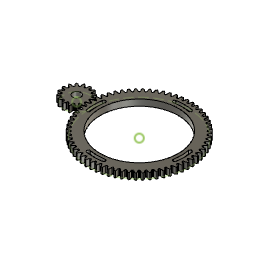
gear use (Autodesk Fusion 360 design; units mm, degrees)
description: Spur Gear; Module: 1.0; Num Teeth: 16; Pressure Angle: 20.0; Backlash: 0.15 mm
description: Spur Gear; Module: 1.0; Num Teeth: 64; Pressure Angle: 20.0; Backlash: 0.15 mm
Autodesk Fusion 360 part; units mm, degrees
(part 1 of 6)
sketch "Sketch1" plane through (0, 0, 0) normal (0, 0, 1) x (1, 0, 0) in component "Spur Gear (16 teeth)"
  circle A0 centre (0, 0) radius 6.7492
  circle A1 centre (0, 0) radius 2.6
  dimension "d41" = 5.2
  measures "d41" diameter of A1
extrude "Extrude1" add sketch "Sketch1" along normal blind 4 makes body 1 in component "Spur Gear (16 teeth)"
sketch "Sketch2" plane through (0, 0, 0) normal (0, 0, 1) x (1, 0, 0) in component "Spur Gear (16 teeth)"
  spline S0 degree 5 poles (7.4734, -0.8132) (7.4777, -0.8137) (7.4864, -0.8145) (7.4993, -0.8154) (7.5167, -0.8158) (7.5384, -0.8154) (7.5601, -0.8143) (7.5819, -0.8127) (7.6037, -0.811) (7.6256, -0.809) (7.6474, -0.8069) (7.6693, -0.8046) (7.6912, -0.8019) (7.7131, -0.799) (7.735, -0.7957) (7.7569, -0.7921) (7.7788, -0.7882) (7.8008, -0.7841) (7.8227, -0.7797) (7.8446, -0.7752) (7.8666, -0.7705) (7.8885, -0.7656) (7.9105, -0.7605) (7.9324, -0.7552) (7.9544, -0.7497) (7.9763, -0.7439) (7.9983, -0.738) (8.0202, -0.7318) (8.0422, -0.7255) (8.0641, -0.719) (8.0861, -0.7124) (8.108, -0.7055) (8.1299, -0.6985) (8.1518, -0.6913) (8.1737, -0.6839) (8.1956, -0.6764) (8.2175, -0.6687) (8.2394, -0.6608) (8.2613, -0.6528) (8.2831, -0.6446) (8.305, -0.6362) (8.3268, -0.6277) (8.3487, -0.619) (8.3705, -0.6102) (8.3923, -0.6012) (8.4141, -0.592) (8.4358, -0.5827) (8.4576, -0.5733) (8.4794, -0.5637) (8.5011, -0.5539) (8.5228, -0.544) (8.5445, -0.534) (8.5662, -0.5238) (8.5878, -0.5135) (8.6095, -0.503) (8.6311, -0.4924) (8.6527, -0.4816) (8.6743, -0.4707) (8.6958, -0.4596) (8.7174, -0.4485) (8.7389, -0.4371) (8.7604, -0.4257) (8.7819, -0.4141) (8.8033, -0.4023) (8.8248, -0.3905) (8.8462, -0.3784) (8.8676, -0.3663) (8.8889, -0.354) (8.9102, -0.3416) (8.9315, -0.3291) (8.9528, -0.3164) (8.9698, -0.3061) (8.9826, -0.2984) (8.9911, -0.2932) (8.9953, -0.2906) knots 0 0 0 0 0 0 0.01428571 0.02857143 0.04285714 0.05714286 0.07142857 0.08571429 0.1 0.11428571 0.12857143 0.14285714 0.15714286 0.17142857 0.18571429 0.2 0.21428571 0.22857143 0.24285714 0.25714286 0.27142857 0.28571429 0.3 0.31428571 0.32857143 0.34285714 0.35714286 0.37142857 0.38571429 0.4 0.41428571 0.42857143 0.44285714 0.45714286 0.47142857 0.48571429 0.5 0.51428571 0.52857143 0.54285714 0.55714286 0.57142857 0.58571429 0.6 0.61428571 0.62857143 0.64285714 0.65714286 0.67142857 0.68571429 0.7 0.71428571 0.72857143 0.74285714 0.75714286 0.77142857 0.78571429 0.8 0.81428571 0.82857143 0.84285714 0.85714286 0.87142857 0.88571429 0.9 0.91428571 0.92857143 0.94285714 0.95714286 0.97142857 0.98571429 1 1 1 1 1 1
  spline S1 degree 5 poles (7.4734, 0.8132) (7.4777, 0.8137) (7.4864, 0.8145) (7.4993, 0.8154) (7.5167, 0.8158) (7.5384, 0.8154) (7.5601, 0.8143) (7.5819, 0.8127) (7.6037, 0.811) (7.6256, 0.809) (7.6474, 0.8069) (7.6693, 0.8046) (7.6912, 0.8019) (7.7131, 0.799) (7.735, 0.7957) (7.7569, 0.7921) (7.7788, 0.7882) (7.8008, 0.7841) (7.8227, 0.7797) (7.8446, 0.7752) (7.8666, 0.7705) (7.8885, 0.7656) (7.9105, 0.7605) (7.9324, 0.7552) (7.9544, 0.7497) (7.9763, 0.7439) (7.9983, 0.738) (8.0202, 0.7318) (8.0422, 0.7255) (8.0641, 0.719) (8.0861, 0.7124) (8.108, 0.7055) (8.1299, 0.6985) (8.1518, 0.6913) (8.1737, 0.6839) (8.1956, 0.6764) (8.2175, 0.6687) (8.2394, 0.6608) (8.2613, 0.6528) (8.2831, 0.6446) (8.305, 0.6362) (8.3268, 0.6277) (8.3487, 0.619) (8.3705, 0.6102) (8.3923, 0.6012) (8.4141, 0.592) (8.4358, 0.5827) (8.4576, 0.5733) (8.4794, 0.5637) (8.5011, 0.5539) (8.5228, 0.544) (8.5445, 0.534) (8.5662, 0.5238) (8.5878, 0.5135) (8.6095, 0.503) (8.6311, 0.4924) (8.6527, 0.4816) (8.6743, 0.4707) (8.6958, 0.4596) (8.7174, 0.4485) (8.7389, 0.4371) (8.7604, 0.4257) (8.7819, 0.4141) (8.8033, 0.4023) (8.8248, 0.3905) (8.8462, 0.3784) (8.8676, 0.3663) (8.8889, 0.354) (8.9102, 0.3416) (8.9315, 0.3291) (8.9528, 0.3164) (8.9698, 0.3061) (8.9826, 0.2984) (8.9911, 0.2932) (8.9953, 0.2906) knots 0 0 0 0 0 0 0.01428571 0.02857143 0.04285714 0.05714286 0.07142857 0.08571429 0.1 0.11428571 0.12857143 0.14285714 0.15714286 0.17142857 0.18571429 0.2 0.21428571 0.22857143 0.24285714 0.25714286 0.27142857 0.28571429 0.3 0.31428571 0.32857143 0.34285714 0.35714286 0.37142857 0.38571429 0.4 0.41428571 0.42857143 0.44285714 0.45714286 0.47142857 0.48571429 0.5 0.51428571 0.52857143 0.54285714 0.55714286 0.57142857 0.58571429 0.6 0.61428571 0.62857143 0.64285714 0.65714286 0.67142857 0.68571429 0.7 0.71428571 0.72857143 0.74285714 0.75714286 0.77142857 0.78571429 0.8 0.81428571 0.82857143 0.84285714 0.85714286 0.87142857 0.88571429 0.9 0.91428571 0.92857143 0.94285714 0.95714286 0.97142857 0.98571429 1 1 1 1 1 1
  arc A0 (8.9953, -0.2906) -> (8.9953, 0.2906) centre (0, 0) ccw
  line L0 (6.6997, -0.7301) -> (7.4734, -0.8132)
  line L1 (6.6997, 0.7301) -> (7.4734, 0.8132)
  line L2 (6.6997, -0.7301) -> (6.6997, 0.7301)
  point P0 (7.58, -0.8128)
  point P1 (7.6876, -0.8023)
  point P2 (7.7958, -0.785)
  point P3 (7.9045, -0.7619)
  point P4 (8.0135, -0.7337)
  point P5 (8.1227, -0.7008)
  point P6 (8.2321, -0.6634)
  point P7 (8.3415, -0.6218)
  point P8 (8.4509, -0.5762)
  point P9 (8.5603, -0.5266)
  point P10 (8.6694, -0.4731)
  point P11 (8.7784, -0.4159)
  point P12 (8.887, -0.3551)
  point P13 (7.58, 0.8128)
  point P14 (7.6876, 0.8023)
  point P15 (7.7958, 0.785)
  point P16 (7.9045, 0.7619)
  point P17 (8.0135, 0.7337)
  point P18 (8.1227, 0.7008)
  point P19 (8.2321, 0.6634)
  point P20 (8.3415, 0.6218)
  point P21 (8.4509, 0.5762)
  point P22 (8.5603, 0.5266)
  point P23 (8.6694, 0.4731)
  point P24 (8.7784, 0.4159)
  point P25 (8.887, 0.3551)
extrude "Extrude2" add sketch "Sketch2" along normal blind 4 bodies 1 in component "Spur Gear (16 teeth)"
fillet "Fillet1" radius 0.5 2 edges at (6.7095, -0.7312, 2) (6.7095, 0.7312, 2) on bodies 1 in component "Spur Gear (16 teeth)"
pattern_circular "C-Pattern1" count 16 over 360 about axis through (0, 0, 0) along (0, 0, 1) of "Extrude2", "Fillet1" in component "Spur Gear (16 teeth)"
sketch "Sketch3" plane through (0, 0, 0) normal (0, 0, 1) x (1, 0, 0) in component "Spur Gear (16 teeth)"
  circle A0 centre (0, 0) radius 8 construction
sketch "Sketch1 (2)" plane through (0, 0, 0) normal (0, 0, 1) x (1, 0, 0) in component "Spur Gear (64 teeth)"
  circle A0 centre (0, 0) radius 30.7492
  circle A1 centre (0, 0) radius 25
extrude "Extrude1'" add sketch "Sketch1 (2)" along normal blind 4 separate body makes body 2 in component "Spur Gear (64 teeth)"
sketch "Sketch2 (2)" plane through (0, 0, 0) normal (0, 0, 1) x (1, 0, 0) in component "Spur Gear (64 teeth)"
  spline S0 degree 5 poles (30.0481, -1.1507) (30.0566, -1.1507) (30.0736, -1.1505) (30.0991, -1.1502) (30.1331, -1.1493) (30.1756, -1.1475) (30.2181, -1.1451) (30.2606, -1.1421) (30.3031, -1.1385) (30.3456, -1.1344) (30.3881, -1.1298) (30.4306, -1.1247) (30.4731, -1.1193) (30.5156, -1.1135) (30.5581, -1.1074) (30.6006, -1.101) (30.643, -1.0942) (30.6855, -1.0872) (30.728, -1.0798) (30.7704, -1.0722) (30.8128, -1.0642) (30.8553, -1.056) (30.8977, -1.0475) (30.9401, -1.0388) (30.9825, -1.0298) (31.0249, -1.0205) (31.0672, -1.011) (31.1096, -1.0012) (31.1519, -0.9913) (31.1943, -0.981) (31.2366, -0.9706) (31.2789, -0.9599) (31.3212, -0.949) (31.3635, -0.9378) (31.4057, -0.9265) (31.448, -0.9149) (31.4902, -0.9032) (31.5324, -0.8912) (31.5746, -0.879) (31.6168, -0.8666) (31.659, -0.854) (31.7011, -0.8413) (31.7433, -0.8283) (31.7854, -0.8151) (31.8275, -0.8017) (31.8696, -0.7882) (31.9116, -0.7744) (31.9537, -0.7605) (31.9957, -0.7464) (32.0377, -0.7321) (32.0797, -0.7176) (32.1216, -0.7029) (32.1636, -0.6881) (32.2055, -0.6731) (32.2474, -0.6579) (32.2893, -0.6425) (32.3312, -0.627) (32.373, -0.6113) (32.4149, -0.5954) (32.4567, -0.5793) (32.4984, -0.5631) (32.5402, -0.5467) (32.5819, -0.5302) (32.6237, -0.5135) (32.6654, -0.4966) (32.707, -0.4796) (32.7487, -0.4624) (32.7903, -0.445) (32.8319, -0.4275) (32.8735, -0.4098) (32.915, -0.392) (32.9483, -0.3776) (32.9732, -0.3667) (32.9898, -0.3594) (32.9981, -0.3558) knots 0 0 0 0 0 0 0.01428571 0.02857143 0.04285714 0.05714286 0.07142857 0.08571429 0.1 0.11428571 0.12857143 0.14285714 0.15714286 0.17142857 0.18571429 0.2 0.21428571 0.22857143 0.24285714 0.25714286 0.27142857 0.28571429 0.3 0.31428571 0.32857143 0.34285714 0.35714286 0.37142857 0.38571429 0.4 0.41428571 0.42857143 0.44285714 0.45714286 0.47142857 0.48571429 0.5 0.51428571 0.52857143 0.54285714 0.55714286 0.57142857 0.58571429 0.6 0.61428571 0.62857143 0.64285714 0.65714286 0.67142857 0.68571429 0.7 0.71428571 0.72857143 0.74285714 0.75714286 0.77142857 0.78571429 0.8 0.81428571 0.82857143 0.84285714 0.85714286 0.87142857 0.88571429 0.9 0.91428571 0.92857143 0.94285714 0.95714286 0.97142857 0.98571429 1 1 1 1 1 1
  spline S1 degree 5 poles (30.0481, 1.1507) (30.0566, 1.1507) (30.0736, 1.1505) (30.0991, 1.1502) (30.1331, 1.1493) (30.1756, 1.1475) (30.2181, 1.1451) (30.2606, 1.1421) (30.3031, 1.1385) (30.3456, 1.1344) (30.3881, 1.1298) (30.4306, 1.1247) (30.4731, 1.1193) (30.5156, 1.1135) (30.5581, 1.1074) (30.6006, 1.101) (30.643, 1.0942) (30.6855, 1.0872) (30.728, 1.0798) (30.7704, 1.0722) (30.8128, 1.0642) (30.8553, 1.056) (30.8977, 1.0475) (30.9401, 1.0388) (30.9825, 1.0298) (31.0249, 1.0205) (31.0672, 1.011) (31.1096, 1.0012) (31.1519, 0.9913) (31.1943, 0.981) (31.2366, 0.9706) (31.2789, 0.9599) (31.3212, 0.949) (31.3635, 0.9378) (31.4057, 0.9265) (31.448, 0.9149) (31.4902, 0.9032) (31.5324, 0.8912) (31.5746, 0.879) (31.6168, 0.8666) (31.659, 0.854) (31.7011, 0.8413) (31.7433, 0.8283) (31.7854, 0.8151) (31.8275, 0.8017) (31.8696, 0.7882) (31.9116, 0.7744) (31.9537, 0.7605) (31.9957, 0.7464) (32.0377, 0.7321) (32.0797, 0.7176) (32.1216, 0.7029) (32.1636, 0.6881) (32.2055, 0.6731) (32.2474, 0.6579) (32.2893, 0.6425) (32.3312, 0.627) (32.373, 0.6113) (32.4149, 0.5954) (32.4567, 0.5793) (32.4984, 0.5631) (32.5402, 0.5467) (32.5819, 0.5302) (32.6237, 0.5135) (32.6654, 0.4966) (32.707, 0.4796) (32.7487, 0.4624) (32.7903, 0.445) (32.8319, 0.4275) (32.8735, 0.4098) (32.915, 0.392) (32.9483, 0.3776) (32.9732, 0.3667) (32.9898, 0.3594) (32.9981, 0.3558) knots 0 0 0 0 0 0 0.01428571 0.02857143 0.04285714 0.05714286 0.07142857 0.08571429 0.1 0.11428571 0.12857143 0.14285714 0.15714286 0.17142857 0.18571429 0.2 0.21428571 0.22857143 0.24285714 0.25714286 0.27142857 0.28571429 0.3 0.31428571 0.32857143 0.34285714 0.35714286 0.37142857 0.38571429 0.4 0.41428571 0.42857143 0.44285714 0.45714286 0.47142857 0.48571429 0.5 0.51428571 0.52857143 0.54285714 0.55714286 0.57142857 0.58571429 0.6 0.61428571 0.62857143 0.64285714 0.65714286 0.67142857 0.68571429 0.7 0.71428571 0.72857143 0.74285714 0.75714286 0.77142857 0.78571429 0.8 0.81428571 0.82857143 0.84285714 0.85714286 0.87142857 0.88571429 0.9 0.91428571 0.92857143 0.94285714 0.95714286 0.97142857 0.98571429 1 1 1 1 1 1
  arc A0 (32.9981, -0.3558) -> (32.9981, 0.3558) centre (0, 0) ccw
  line L0 (30.0481, 1.1507) -> (30.0481, -1.1507)
  point P0 (30.2579, -1.1422)
  point P1 (30.4681, -1.1198)
  point P2 (30.6787, -1.0883)
  point P3 (30.8894, -1.0491)
  point P4 (31.1004, -1.0033)
  point P5 (31.3114, -0.9515)
  point P6 (31.5224, -0.894)
  point P7 (31.7335, -0.8313)
  point P8 (31.9445, -0.7635)
  point P9 (32.1555, -0.6909)
  point P10 (32.3664, -0.6137)
  point P11 (32.5771, -0.5321)
  point P12 (32.7877, -0.446)
  point P13 (30.2579, 1.1422)
  point P14 (30.4681, 1.1198)
  point P15 (30.6787, 1.0883)
  point P16 (30.8894, 1.0491)
  point P17 (31.1004, 1.0033)
  point P18 (31.3114, 0.9515)
  point P19 (31.5224, 0.894)
  point P20 (31.7335, 0.8313)
  point P21 (31.9445, 0.7635)
  point P22 (32.1555, 0.6909)
  point P23 (32.3664, 0.6137)
  point P24 (32.5771, 0.5321)
  point P25 (32.7877, 0.446)
extrude "Extrude2'" add sketch "Sketch2 (2)" along normal blind 4 bodies 2 in component "Spur Gear (64 teeth)"
fillet "Fillet1'" radius 0.5 2 edges at (30.7303, 1.0794, 2) (30.7303, -1.0794, 2) on bodies 2 in component "Spur Gear (64 teeth)"
pattern_circular "C-Pattern1'" count 64 over 360 about axis through (0, 0, -0.0002) along (0, 0, 1) of "Extrude2'", "Fillet1'" in component "Spur Gear (64 teeth)"
sketch "Sketch3 (2)" plane through (0, 0, 0) normal (0, 0, 1) x (1, 0, 0) in component "Spur Gear (64 teeth)"
  circle A0 centre (0, 0) radius 32 construction
sketch "Sketch1 (3)" plane through (0, 0, 0) normal (0, 0, 1) x (1, 0, 0)
  circle A0 centre (0, 0) radius 10
  circle A1 centre (40, 0) radius 33.936
  line L0 (19.6927, 27.1894) -> (-5.984, 8.012)
  line L1 (0, 0) -> (40, 0) construction
  line L2 (19.6927, -27.1894) -> (-5.984, -8.012)
  point P0 (40, 0)
  constraint coincident A0.centre L1.start
  constraint tangent A1 L0
  constraint tangent A0 L0
  constraint coincident P0 A1.centre
  constraint coincident A1 L0.start
  constraint coincident A0 L0.end
  constraint symmetric L0.start L1 L2.start
  constraint symmetric L0.end L1 L2.end
sketch "Sketch3 (3)" plane through (0, 0, 4) normal (0, 0, 1) x (-1, 0, 0)
  arc A0 (-70.5976, 3.0494) -> (-70.6059, 2.9651) centre (-40, 0) ccw
  spline S0 degree 3 poles (-71.0146, 2.5213) (-70.9505, 2.5329) (-70.8893, 2.5569) (-70.7796, 2.627) (-70.7321, 2.6724) (-70.6698, 2.7609) (-70.6497, 2.7992) (-70.6197, 2.88) (-70.6101, 2.9222) (-70.6059, 2.9651) knots 0 0 0 0 0.019532 0.019532 0.039064 0.039064 0.051994 0.051994 0.064924 0.064924 0.064924 0.064924
  spline S1 degree 5 poles (-71.0146, 2.5213) (-71.0164, 2.521) (-71.0267, 2.5191) (-71.0456, 2.5157) (-71.0731, 2.5105) (-71.1091, 2.5037) (-71.1519, 2.4953) (-71.1947, 2.4867) (-71.2374, 2.4779) (-71.2802, 2.4688) (-71.323, 2.4596) (-71.3657, 2.4501) (-71.4085, 2.4404) (-71.4512, 2.4305) (-71.494, 2.4204) (-71.5367, 2.4101) (-71.5795, 2.3996) (-71.6222, 2.3889) (-71.6649, 2.3779) (-71.7076, 2.3668) (-71.7503, 2.3555) (-71.793, 2.3441) (-71.8357, 2.3324) (-71.8784, 2.3205) (-71.921, 2.3085) (-71.9637, 2.2962) (-72.0063, 2.2838) (-72.049, 2.2712) (-72.0916, 2.2585) (-72.1342, 2.2455) (-72.1768, 2.2324) (-72.2194, 2.2191) (-72.262, 2.2056) (-72.3045, 2.192) (-72.3471, 2.1781) (-72.3896, 2.1641) (-72.4321, 2.15) (-72.4746, 2.1357) (-72.5171, 2.1212) (-72.5596, 2.1065) (-72.6021, 2.0917) (-72.6446, 2.0767) (-72.687, 2.0616) (-72.7294, 2.0463) (-72.7718, 2.0308) (-72.8142, 2.0152) (-72.8566, 1.9994) (-72.8905, 1.9866) (-72.9159, 1.977) (-72.9328, 1.9705) (-72.9413, 1.9673) knots 0.354152 0.354152 0.354152 0.354152 0.354152 0.354152 0.357143 0.371429 0.385714 0.4 0.414286 0.428571 0.442857 0.457143 0.471429 0.485714 0.5 0.514286 0.528571 0.542857 0.557143 0.571429 0.585714 0.6 0.614286 0.628571 0.642857 0.657143 0.671429 0.685714 0.7 0.714286 0.728571 0.742857 0.757143 0.771429 0.785714 0.8 0.814286 0.828571 0.842857 0.857143 0.871429 0.885714 0.9 0.914286 0.928571 0.942857 0.957143 0.971429 0.985714 1 1 1 1 1 1
  arc A1 (-72.9413, 1.9673) -> (-72.9761, 1.2566) centre (-40, 0) ccw
  spline S2 degree 5 poles (-72.9761, 1.2566) (-72.968, 1.2525) (-72.9517, 1.2445) (-72.9274, 1.2324) (-72.8949, 1.2164) (-72.8543, 1.1966) (-72.8136, 1.1769) (-72.7729, 1.1573) (-72.7322, 1.138) (-72.6914, 1.1188) (-72.6506, 1.0997) (-72.6098, 1.0808) (-72.5689, 1.0621) (-72.5281, 1.0435) (-72.4872, 1.0251) (-72.4462, 1.0069) (-72.4052, 0.9888) (-72.3642, 0.9709) (-72.3232, 0.9531) (-72.2822, 0.9356) (-72.2411, 0.9182) (-72.2, 0.901) (-72.1588, 0.8839) (-72.1176, 0.867) (-72.0764, 0.8503) (-72.0352, 0.8338) (-71.9939, 0.8175) (-71.9527, 0.8013) (-71.9113, 0.7854) (-71.87, 0.7696) (-71.8286, 0.754) (-71.7872, 0.7386) (-71.7458, 0.7234) (-71.7044, 0.7083) (-71.6629, 0.6935) (-71.6214, 0.6789) (-71.5799, 0.6644) (-71.5383, 0.6502) (-71.4967, 0.6362) (-71.4551, 0.6224) (-71.4135, 0.6088) (-71.3718, 0.5954) (-71.3302, 0.5822) (-71.2885, 0.5692) (-71.2467, 0.5565) (-71.205, 0.544) (-71.1698, 0.5336) (-71.143, 0.5259) (-71.1245, 0.5206) (-71.1144, 0.5177) (-71.1126, 0.5172) knots -1 -1 -1 -1 -1 -1 -0.985714 -0.971429 -0.957143 -0.942857 -0.928571 -0.914286 -0.9 -0.885714 -0.871429 -0.857143 -0.842857 -0.828571 -0.814286 -0.8 -0.785714 -0.771429 -0.757143 -0.742857 -0.728571 -0.714286 -0.7 -0.685714 -0.671429 -0.657143 -0.642857 -0.628571 -0.614286 -0.6 -0.585714 -0.571429 -0.557143 -0.542857 -0.528571 -0.514286 -0.5 -0.485714 -0.471429 -0.457143 -0.442857 -0.428571 -0.414286 -0.4 -0.385714 -0.371429 -0.357143 -0.354152 -0.354152 -0.354152 -0.354152 -0.354152 -0.354152
  spline S3 degree 3 poles (-70.7492, 0.0357) (-70.7491, 0.1008) (-70.7617, 0.1653) (-70.811, 0.2858) (-70.8472, 0.3407) (-70.9231, 0.4178) (-70.9572, 0.4444) (-71.0314, 0.4884) (-71.0712, 0.5054) (-71.1126, 0.5172) knots 0 0 0 0 0.019532 0.019532 0.039064 0.039064 0.051994 0.051994 0.064924 0.064924 0.064924 0.064924
  arc A2 (-70.7492, 0.0357) -> (-70.7492, -0.0491) centre (-40, 0) ccw
  spline S4 degree 3 poles (-71.1124, -0.5308) (-71.0498, -0.513) (-70.9912, -0.4831) (-70.8889, -0.4026) (-70.846, -0.3527) (-70.7928, -0.2586) (-70.7765, -0.2185) (-70.7546, -0.1351) (-70.7491, -0.0922) (-70.7492, -0.0491) knots 0 0 0 0 0.019532 0.019532 0.039064 0.039064 0.051994 0.051994 0.064924 0.064924 0.064924 0.064924
  spline S5 degree 5 poles (-71.1124, -0.5308) (-71.1141, -0.5313) (-71.1242, -0.5342) (-71.1427, -0.5395) (-71.1696, -0.5472) (-71.2047, -0.5576) (-71.2465, -0.5701) (-71.2882, -0.5829) (-71.3299, -0.5959) (-71.3716, -0.6091) (-71.4132, -0.6225) (-71.4549, -0.6361) (-71.4965, -0.6499) (-71.538, -0.664) (-71.5796, -0.6782) (-71.6211, -0.6927) (-71.6626, -0.7073) (-71.7041, -0.7222) (-71.7455, -0.7372) (-71.7869, -0.7524) (-71.8283, -0.7679) (-71.8697, -0.7835) (-71.911, -0.7993) (-71.9523, -0.8153) (-71.9936, -0.8314) (-72.0348, -0.8478) (-72.0761, -0.8643) (-72.1173, -0.8811) (-72.1584, -0.8979) (-72.1996, -0.915) (-72.2407, -0.9322) (-72.2817, -0.9497) (-72.3228, -0.9672) (-72.3638, -0.985) (-72.4048, -1.0029) (-72.4458, -1.021) (-72.4867, -1.0393) (-72.5276, -1.0577) (-72.5685, -1.0763) (-72.6093, -1.095) (-72.6501, -1.1139) (-72.6909, -1.133) (-72.7317, -1.1522) (-72.7724, -1.1716) (-72.8131, -1.1912) (-72.8537, -1.2109) (-72.8944, -1.2308) (-72.9268, -1.2468) (-72.9512, -1.2588) (-72.9674, -1.2669) (-72.9755, -1.271) knots 0.354152 0.354152 0.354152 0.354152 0.354152 0.354152 0.357143 0.371429 0.385714 0.4 0.414286 0.428571 0.442857 0.457143 0.471429 0.485714 0.5 0.514286 0.528571 0.542857 0.557143 0.571429 0.585714 0.6 0.614286 0.628571 0.642857 0.657143 0.671429 0.685714 0.7 0.714286 0.728571 0.742857 0.757143 0.771429 0.785714 0.8 0.814286 0.828571 0.842857 0.857143 0.871429 0.885714 0.9 0.914286 0.928571 0.942857 0.957143 0.971429 0.985714 1 1 1 1 1 1
  arc A3 (-72.9755, -1.271) -> (-72.9404, -1.9817) centre (-40, 0) ccw
  spline S6 degree 5 poles (-72.9404, -1.9817) (-72.932, -1.9849) (-72.915, -1.9914) (-72.8896, -2.001) (-72.8557, -2.0137) (-72.8133, -2.0295) (-72.7709, -2.0451) (-72.7285, -2.0605) (-72.6861, -2.0758) (-72.6436, -2.091) (-72.6012, -2.1059) (-72.5587, -2.1207) (-72.5162, -2.1354) (-72.4737, -2.1498) (-72.4312, -2.1641) (-72.3887, -2.1783) (-72.3461, -2.1922) (-72.3036, -2.206) (-72.261, -2.2197) (-72.2184, -2.2331) (-72.1758, -2.2464) (-72.1332, -2.2595) (-72.0906, -2.2725) (-72.048, -2.2852) (-72.0053, -2.2978) (-71.9627, -2.3102) (-71.92, -2.3224) (-71.8773, -2.3344) (-71.8347, -2.3463) (-71.792, -2.3579) (-71.7493, -2.3694) (-71.7066, -2.3807) (-71.6639, -2.3918) (-71.6211, -2.4027) (-71.5784, -2.4133) (-71.5357, -2.4238) (-71.4929, -2.4341) (-71.4502, -2.4442) (-71.4074, -2.4541) (-71.3647, -2.4638) (-71.3219, -2.4732) (-71.2791, -2.4825) (-71.2364, -2.4915) (-71.1936, -2.5003) (-71.1508, -2.5089) (-71.108, -2.5173) (-71.072, -2.5241) (-71.0445, -2.5292) (-71.0256, -2.5326) (-71.0153, -2.5345) (-71.0135, -2.5348) knots -1 -1 -1 -1 -1 -1 -0.985714 -0.971429 -0.957143 -0.942857 -0.928571 -0.914286 -0.9 -0.885714 -0.871429 -0.857143 -0.842857 -0.828571 -0.814286 -0.8 -0.785714 -0.771429 -0.757143 -0.742857 -0.728571 -0.714286 -0.7 -0.685714 -0.671429 -0.657143 -0.642857 -0.628571 -0.614286 -0.6 -0.585714 -0.571429 -0.557143 -0.542857 -0.528571 -0.514286 -0.5 -0.485714 -0.471429 -0.457143 -0.442857 -0.428571 -0.414286 -0.4 -0.385714 -0.371429 -0.357143 -0.354152 -0.354152 -0.354152 -0.354152 -0.354152 -0.354152
  spline S7 degree 3 poles (-70.6046, -2.9785) (-70.6109, -2.9137) (-70.6298, -2.8507) (-70.6907, -2.7356) (-70.7321, -2.6845) (-70.8152, -2.6153) (-70.8517, -2.5921) (-70.9298, -2.5556) (-70.9711, -2.5425) (-71.0135, -2.5348) knots 0 0 0 0 0.019532 0.019532 0.039064 0.039064 0.051994 0.051994 0.064924 0.064924 0.064924 0.064924
  arc A4 (-70.6046, -2.9785) -> (-70.5963, -3.0628) centre (-40, 0) ccw
  spline S8 degree 3 poles (-70.9105, -3.5778) (-70.85, -3.5539) (-70.7946, -3.5185) (-70.7007, -3.4283) (-70.6629, -3.3745) (-70.6191, -3.2755) (-70.6069, -3.234) (-70.5933, -3.1489) (-70.592, -3.1057) (-70.5963, -3.0628) knots 0 0 0 0 0.019532 0.019532 0.039064 0.039064 0.051994 0.051994 0.064924 0.064924 0.064924 0.064924
  spline S9 degree 5 poles (-70.9105, -3.5778) (-70.9122, -3.5785) (-70.922, -3.5823) (-70.9399, -3.5894) (-70.9658, -3.5998) (-70.9998, -3.6135) (-71.0401, -3.6301) (-71.0804, -3.6469) (-71.1206, -3.6639) (-71.1608, -3.6811) (-71.201, -3.6985) (-71.241, -3.7161) (-71.2811, -3.734) (-71.3211, -3.752) (-71.361, -3.7703) (-71.4009, -3.7887) (-71.4408, -3.8074) (-71.4806, -3.8262) (-71.5204, -3.8453) (-71.5601, -3.8645) (-71.5998, -3.8839) (-71.6394, -3.9035) (-71.679, -3.9233) (-71.7185, -3.9432) (-71.758, -3.9634) (-71.7975, -3.9837) (-71.8369, -4.0042) (-71.8762, -4.0248) (-71.9156, -4.0457) (-71.9548, -4.0667) (-71.994, -4.0879) (-72.0332, -4.1093) (-72.0723, -4.1308) (-72.1114, -4.1525) (-72.1505, -4.1743) (-72.1895, -4.1963) (-72.2284, -4.2185) (-72.2673, -4.2409) (-72.3062, -4.2634) (-72.345, -4.286) (-72.3837, -4.3089) (-72.4224, -4.3318) (-72.4611, -4.355) (-72.4997, -4.3783) (-72.5383, -4.4017) (-72.5768, -4.4253) (-72.6153, -4.449) (-72.6461, -4.4682) (-72.6691, -4.4826) (-72.6845, -4.4922) (-72.6922, -4.497) knots 0.354152 0.354152 0.354152 0.354152 0.354152 0.354152 0.357143 0.371429 0.385714 0.4 0.414286 0.428571 0.442857 0.457143 0.471429 0.485714 0.5 0.514286 0.528571 0.542857 0.557143 0.571429 0.585714 0.6 0.614286 0.628571 0.642857 0.657143 0.671429 0.685714 0.7 0.714286 0.728571 0.742857 0.757143 0.771429 0.785714 0.8 0.814286 0.828571 0.842857 0.857143 0.871429 0.885714 0.9 0.914286 0.928571 0.942857 0.957143 0.971429 0.985714 1 1 1 1 1 1
  arc A5 (-72.6922, -4.497) -> (-72.5876, -5.2009) centre (-40, 0) ccw
  spline S10 degree 5 poles (-72.5876, -5.2009) (-72.5788, -5.2033) (-72.5614, -5.208) (-72.5351, -5.2151) (-72.5001, -5.2245) (-72.4564, -5.236) (-72.4127, -5.2474) (-72.369, -5.2586) (-72.3252, -5.2696) (-72.2815, -5.2805) (-72.2378, -5.2913) (-72.1941, -5.3018) (-72.1503, -5.3122) (-72.1066, -5.3225) (-72.0629, -5.3325) (-72.0192, -5.3424) (-71.9755, -5.3522) (-71.9318, -5.3617) (-71.8881, -5.3711) (-71.8444, -5.3803) (-71.8007, -5.3894) (-71.757, -5.3983) (-71.7133, -5.4069) (-71.6697, -5.4155) (-71.626, -5.4238) (-71.5823, -5.432) (-71.5387, -5.4399) (-71.495, -5.4477) (-71.4514, -5.4553) (-71.4078, -5.4627) (-71.3642, -5.47) (-71.3206, -5.477) (-71.277, -5.4838) (-71.2334, -5.4905) (-71.1898, -5.4969) (-71.1462, -5.5032) (-71.1027, -5.5093) (-71.0592, -5.5151) (-71.0156, -5.5207) (-70.9721, -5.5262) (-70.9287, -5.5314) (-70.8852, -5.5364) (-70.8417, -5.5412) (-70.7983, -5.5458) (-70.7549, -5.5501) (-70.7115, -5.5543) (-70.675, -5.5575) (-70.6471, -5.5599) (-70.628, -5.5615) (-70.6175, -5.5623) (-70.6157, -5.5625) knots -1 -1 -1 -1 -1 -1 -0.985714 -0.971429 -0.957143 -0.942857 -0.928571 -0.914286 -0.9 -0.885714 -0.871429 -0.857143 -0.842857 -0.828571 -0.814286 -0.8 -0.785714 -0.771429 -0.757143 -0.742857 -0.728571 -0.714286 -0.7 -0.685714 -0.671429 -0.657143 -0.642857 -0.628571 -0.614286 -0.6 -0.585714 -0.571429 -0.557143 -0.542857 -0.528571 -0.514286 -0.5 -0.485714 -0.471429 -0.457143 -0.442857 -0.428571 -0.414286 -0.4 -0.385714 -0.371429 -0.357143 -0.354152 -0.354152 -0.354152 -0.354152 -0.354152 -0.354152
  spline S11 degree 3 poles (-70.1653, -5.9639) (-70.1779, -5.9) (-70.2029, -5.8392) (-70.2748, -5.7306) (-70.321, -5.6839) (-70.4105, -5.6231) (-70.4491, -5.6036) (-70.5304, -5.5749) (-70.5727, -5.5659) (-70.6157, -5.5625) knots 0 0 0 0 0.019532 0.019532 0.039064 0.039064 0.051994 0.051994 0.064924 0.064924 0.064924 0.064924
  arc A6 (-70.1653, -5.9639) -> (-70.1488, -6.047) centre (-40, 0) ccw
  spline S12 degree 3 poles (-70.411, -6.5903) (-70.3531, -6.5606) (-70.3015, -6.5199) (-70.2168, -6.421) (-70.1845, -6.3637) (-70.1506, -6.261) (-70.1425, -6.2185) (-70.1373, -6.1324) (-70.1403, -6.0892) (-70.1488, -6.047) knots 0 0 0 0 0.019532 0.019532 0.039064 0.039064 0.051994 0.051994 0.064924 0.064924 0.064924 0.064924
  spline S13 degree 5 poles (-70.411, -6.5903) (-70.4126, -6.5912) (-70.422, -6.5959) (-70.4391, -6.6047) (-70.4639, -6.6176) (-70.4964, -6.6346) (-70.5349, -6.6551) (-70.5733, -6.6757) (-70.6117, -6.6966) (-70.65, -6.7176) (-70.6882, -6.7389) (-70.7264, -6.7604) (-70.7645, -6.7821) (-70.8025, -6.804) (-70.8405, -6.8261) (-70.8784, -6.8483) (-70.9162, -6.8708) (-70.954, -6.8934) (-70.9917, -6.9163) (-71.0293, -6.9393) (-71.0669, -6.9625) (-71.1045, -6.9859) (-71.1419, -7.0095) (-71.1793, -7.0332) (-71.2166, -7.0571) (-71.2539, -7.0812) (-71.2911, -7.1055) (-71.3282, -7.1299) (-71.3653, -7.1545) (-71.4023, -7.1792) (-71.4393, -7.2042) (-71.4762, -7.2293) (-71.513, -7.2545) (-71.5498, -7.2799) (-71.5865, -7.3055) (-71.6231, -7.3313) (-71.6597, -7.3571) (-71.6963, -7.3832) (-71.7327, -7.4094) (-71.7691, -7.4358) (-71.8055, -7.4623) (-71.8417, -7.4889) (-71.8779, -7.5157) (-71.9141, -7.5427) (-71.9502, -7.5698) (-71.9862, -7.5971) (-72.0222, -7.6245) (-72.0509, -7.6465) (-72.0724, -7.6631) (-72.0868, -7.6742) (-72.0939, -7.6798) knots 0.354152 0.354152 0.354152 0.354152 0.354152 0.354152 0.357143 0.371429 0.385714 0.4 0.414286 0.428571 0.442857 0.457143 0.471429 0.485714 0.5 0.514286 0.528571 0.542857 0.557143 0.571429 0.585714 0.6 0.614286 0.628571 0.642857 0.657143 0.671429 0.685714 0.7 0.714286 0.728571 0.742857 0.757143 0.771429 0.785714 0.8 0.814286 0.828571 0.842857 0.857143 0.871429 0.885714 0.9 0.914286 0.928571 0.942857 0.957143 0.971429 0.985714 1 1 1 1 1 1
  arc A7 (-72.0939, -7.6798) -> (-71.9209, -8.37) centre (-40, 0) ccw
  spline S14 degree 5 poles (-71.9209, -8.37) (-71.912, -8.3715) (-71.8941, -8.3745) (-71.8673, -8.379) (-71.8316, -8.3849) (-71.7869, -8.3921) (-71.7423, -8.3991) (-71.6977, -8.406) (-71.6531, -8.4127) (-71.6085, -8.4192) (-71.5639, -8.4256) (-71.5194, -8.4319) (-71.4748, -8.4379) (-71.4303, -8.4438) (-71.3858, -8.4496) (-71.3414, -8.4551) (-71.2969, -8.4605) (-71.2525, -8.4658) (-71.2081, -8.4708) (-71.1637, -8.4757) (-71.1193, -8.4804) (-71.075, -8.485) (-71.0306, -8.4894) (-70.9863, -8.4936) (-70.9421, -8.4976) (-70.8978, -8.5014) (-70.8536, -8.5051) (-70.8094, -8.5085) (-70.7652, -8.5118) (-70.7211, -8.5149) (-70.677, -8.5178) (-70.6329, -8.5206) (-70.5888, -8.5231) (-70.5448, -8.5255) (-70.5008, -8.5276) (-70.4569, -8.5296) (-70.4129, -8.5313) (-70.369, -8.5329) (-70.3252, -8.5342) (-70.2813, -8.5354) (-70.2376, -8.5363) (-70.1938, -8.537) (-70.1501, -8.5375) (-70.1064, -8.5378) (-70.0628, -8.5379) (-70.0192, -8.5378) (-69.9825, -8.5375) (-69.9546, -8.5371) (-69.9354, -8.5368) (-69.9249, -8.5366) (-69.9231, -8.5366) knots -1 -1 -1 -1 -1 -1 -0.985714 -0.971429 -0.957143 -0.942857 -0.928571 -0.914286 -0.9 -0.885714 -0.871429 -0.857143 -0.842857 -0.828571 -0.814286 -0.8 -0.785714 -0.771429 -0.757143 -0.742857 -0.728571 -0.714286 -0.7 -0.685714 -0.671429 -0.657143 -0.642857 -0.628571 -0.614286 -0.6 -0.585714 -0.571429 -0.557143 -0.542857 -0.528571 -0.514286 -0.5 -0.485714 -0.471429 -0.457143 -0.442857 -0.428571 -0.414286 -0.4 -0.385714 -0.371429 -0.357143 -0.354152 -0.354152 -0.354152 -0.354152 -0.354152 -0.354152
  spline S15 degree 3 poles (-69.4355, -8.8919) (-69.4543, -8.8296) (-69.4851, -8.7715) (-69.5673, -8.6705) (-69.6178, -8.6285) (-69.7129, -8.5767) (-69.7532, -8.5611) (-69.837, -8.5406) (-69.88, -8.5358) (-69.9231, -8.5366) knots 0 0 0 0 0.019532 0.019532 0.039064 0.039064 0.051994 0.051994 0.064924 0.064924 0.064924 0.064924
  arc A8 (-69.4355, -8.8919) -> (-69.4109, -8.973) centre (-40, 0) ccw
  spline S16 degree 3 poles (-69.6186, -9.5394) (-69.5639, -9.5042) (-69.5165, -9.4586) (-69.4419, -9.3518) (-69.4154, -9.2917) (-69.3918, -9.1861) (-69.3878, -9.143) (-69.3911, -9.0569) (-69.3983, -9.0142) (-69.4109, -8.973) knots 0 0 0 0 0.019532 0.019532 0.039064 0.039064 0.051994 0.051994 0.064924 0.064924 0.064924 0.064924
  spline S17 degree 5 poles (-69.6186, -9.5394) (-69.6201, -9.5404) (-69.629, -9.5461) (-69.6451, -9.5565) (-69.6685, -9.5717) (-69.6992, -9.5918) (-69.7355, -9.6159) (-69.7717, -9.6403) (-69.8079, -9.6648) (-69.8439, -9.6895) (-69.8799, -9.7144) (-69.9158, -9.7396) (-69.9516, -9.7649) (-69.9873, -9.7904) (-70.0229, -9.8161) (-70.0584, -9.842) (-70.0939, -9.868) (-70.1293, -9.8943) (-70.1646, -9.9207) (-70.1998, -9.9473) (-70.2349, -9.9741) (-70.2699, -10.001) (-70.3049, -10.0281) (-70.3398, -10.0554) (-70.3746, -10.0829) (-70.4093, -10.1105) (-70.444, -10.1383) (-70.4785, -10.1663) (-70.513, -10.1944) (-70.5474, -10.2226) (-70.5818, -10.2511) (-70.616, -10.2797) (-70.6502, -10.3084) (-70.6843, -10.3373) (-70.7183, -10.3664) (-70.7523, -10.3956) (-70.7862, -10.4249) (-70.8199, -10.4544) (-70.8537, -10.4841) (-70.8873, -10.5139) (-70.9209, -10.5438) (-70.9544, -10.5739) (-70.9878, -10.6041) (-71.0211, -10.6345) (-71.0544, -10.665) (-71.0876, -10.6957) (-71.1207, -10.7265) (-71.1471, -10.7512) (-71.1669, -10.7699) (-71.1801, -10.7823) (-71.1867, -10.7885) knots 0.354152 0.354152 0.354152 0.354152 0.354152 0.354152 0.357143 0.371429 0.385714 0.4 0.414286 0.428571 0.442857 0.457143 0.471429 0.485714 0.5 0.514286 0.528571 0.542857 0.557143 0.571429 0.585714 0.6 0.614286 0.628571 0.642857 0.657143 0.671429 0.685714 0.7 0.714286 0.728571 0.742857 0.757143 0.771429 0.785714 0.8 0.814286 0.828571 0.842857 0.857143 0.871429 0.885714 0.9 0.914286 0.928571 0.942857 0.957143 0.971429 0.985714 1 1 1 1 1 1
  arc A9 (-71.1867, -10.7885) -> (-70.9468, -11.4585) centre (-40, 0) ccw
  spline S18 degree 5 poles (-70.9468, -11.4585) (-70.9377, -11.4591) (-70.9197, -11.4603) (-70.8926, -11.4622) (-70.8564, -11.4645) (-70.8113, -11.4673) (-70.7662, -11.4699) (-70.7211, -11.4724) (-70.6761, -11.4747) (-70.6311, -11.4769) (-70.5861, -11.4789) (-70.5411, -11.4807) (-70.4962, -11.4824) (-70.4513, -11.4839) (-70.4065, -11.4852) (-70.3617, -11.4864) (-70.3169, -11.4874) (-70.2722, -11.4883) (-70.2275, -11.489) (-70.1829, -11.4895) (-70.1382, -11.4898) (-70.0937, -11.49) (-70.0491, -11.49) (-70.0046, -11.4898) (-69.9602, -11.4895) (-69.9158, -11.489) (-69.8714, -11.4883) (-69.8271, -11.4874) (-69.7828, -11.4864) (-69.7386, -11.4851) (-69.6944, -11.4837) (-69.6502, -11.4821) (-69.6061, -11.4803) (-69.5621, -11.4783) (-69.5181, -11.4762) (-69.4742, -11.4738) (-69.4303, -11.4712) (-69.3864, -11.4685) (-69.3426, -11.4655) (-69.2989, -11.4624) (-69.2553, -11.459) (-69.2116, -11.4554) (-69.1681, -11.4517) (-69.1246, -11.4477) (-69.0812, -11.4435) (-69.0378, -11.4391) (-69.0013, -11.4351) (-68.9736, -11.432) (-68.9545, -11.4299) (-68.944, -11.4286) (-68.9422, -11.4284) knots -1 -1 -1 -1 -1 -1 -0.985714 -0.971429 -0.957143 -0.942857 -0.928571 -0.914286 -0.9 -0.885714 -0.871429 -0.857143 -0.842857 -0.828571 -0.814286 -0.8 -0.785714 -0.771429 -0.757143 -0.742857 -0.728571 -0.714286 -0.7 -0.685714 -0.671429 -0.657143 -0.642857 -0.628571 -0.614286 -0.6 -0.585714 -0.571429 -0.557143 -0.542857 -0.528571 -0.514286 -0.5 -0.485714 -0.471429 -0.457143 -0.442857 -0.428571 -0.414286 -0.4 -0.385714 -0.371429 -0.357143 -0.354152 -0.354152 -0.354152 -0.354152 -0.354152 -0.354152
  spline S19 degree 3 poles (-68.4222, -11.7343) (-68.447, -11.6741) (-68.4834, -11.6193) (-68.5751, -11.5268) (-68.6295, -11.49) (-68.7291, -11.4478) (-68.7708, -11.4362) (-68.8562, -11.424) (-68.8994, -11.4234) (-68.9422, -11.4284) knots 0 0 0 0 0.019532 0.019532 0.039064 0.039064 0.051994 0.051994 0.064924 0.064924 0.064924 0.064924
  arc A10 (-68.4222, -11.7343) -> (-68.3897, -11.8125) centre (-40, 0) ccw
  spline S20 degree 3 poles (-68.541, -12.3966) (-68.4899, -12.3562) (-68.4473, -12.3062) (-68.3835, -12.1926) (-68.363, -12.1302) (-68.3499, -12.0228) (-68.3502, -11.9795) (-68.3618, -11.8941) (-68.3732, -11.8523) (-68.3897, -11.8125) knots 0 0 0 0 0.019532 0.019532 0.039064 0.039064 0.051994 0.051994 0.064924 0.064924 0.064924 0.064924
  spline S21 degree 5 poles (-68.541, -12.3966) (-68.5424, -12.3977) (-68.5506, -12.4042) (-68.5657, -12.4162) (-68.5875, -12.4337) (-68.616, -12.4567) (-68.6498, -12.4842) (-68.6835, -12.512) (-68.717, -12.5399) (-68.7505, -12.5681) (-68.7838, -12.5964) (-68.8171, -12.6249) (-68.8502, -12.6536) (-68.8832, -12.6825) (-68.9162, -12.7116) (-68.949, -12.7408) (-68.9817, -12.7702) (-69.0144, -12.7998) (-69.0469, -12.8296) (-69.0793, -12.8595) (-69.1117, -12.8896) (-69.1439, -12.9198) (-69.176, -12.9503) (-69.2081, -12.9808) (-69.24, -13.0116) (-69.2719, -13.0425) (-69.3036, -13.0735) (-69.3353, -13.1047) (-69.3669, -13.1361) (-69.3984, -13.1676) (-69.4297, -13.1993) (-69.461, -13.2311) (-69.4922, -13.263) (-69.5233, -13.2951) (-69.5543, -13.3274) (-69.5853, -13.3598) (-69.6161, -13.3923) (-69.6468, -13.425) (-69.6775, -13.4578) (-69.708, -13.4907) (-69.7385, -13.5238) (-69.7689, -13.557) (-69.7992, -13.5904) (-69.8294, -13.6239) (-69.8595, -13.6575) (-69.8895, -13.6913) (-69.9194, -13.7252) (-69.9433, -13.7524) (-69.9612, -13.7729) (-69.9731, -13.7866) (-69.979, -13.7934) knots 0.354152 0.354152 0.354152 0.354152 0.354152 0.354152 0.357143 0.371429 0.385714 0.4 0.414286 0.428571 0.442857 0.457143 0.471429 0.485714 0.5 0.514286 0.528571 0.542857 0.557143 0.571429 0.585714 0.6 0.614286 0.628571 0.642857 0.657143 0.671429 0.685714 0.7 0.714286 0.728571 0.742857 0.757143 0.771429 0.785714 0.8 0.814286 0.828571 0.842857 0.857143 0.871429 0.885714 0.9 0.914286 0.928571 0.942857 0.957143 0.971429 0.985714 1 1 1 1 1 1
  arc A11 (-69.979, -13.7934) -> (-69.6746, -14.4366) centre (-40, 0) ccw
  spline S22 degree 5 poles (-69.6746, -14.4366) (-69.6656, -14.4363) (-69.6475, -14.4358) (-69.6203, -14.435) (-69.5841, -14.4338) (-69.5389, -14.4321) (-69.4938, -14.4303) (-69.4487, -14.4284) (-69.4036, -14.4262) (-69.3586, -14.424) (-69.3137, -14.4215) (-69.2688, -14.419) (-69.2239, -14.4162) (-69.1791, -14.4133) (-69.1343, -14.4103) (-69.0896, -14.4071) (-69.045, -14.4037) (-69.0004, -14.4002) (-68.9558, -14.3965) (-68.9113, -14.3926) (-68.8669, -14.3886) (-68.8225, -14.3844) (-68.7782, -14.38) (-68.7339, -14.3755) (-68.6897, -14.3708) (-68.6456, -14.3659) (-68.6015, -14.3609) (-68.5575, -14.3557) (-68.5135, -14.3503) (-68.4696, -14.3447) (-68.4258, -14.339) (-68.382, -14.333) (-68.3383, -14.3269) (-68.2947, -14.3206) (-68.2511, -14.3142) (-68.2076, -14.3075) (-68.1642, -14.3007) (-68.1208, -14.2936) (-68.0775, -14.2864) (-68.0343, -14.279) (-67.9912, -14.2713) (-67.9482, -14.2635) (-67.9052, -14.2555) (-67.8623, -14.2473) (-67.8195, -14.2388) (-67.7767, -14.2302) (-67.7409, -14.2227) (-67.7135, -14.2169) (-67.6947, -14.2129) (-67.6845, -14.2106) (-67.6827, -14.2102) knots -1 -1 -1 -1 -1 -1 -0.985714 -0.971429 -0.957143 -0.942857 -0.928571 -0.914286 -0.9 -0.885714 -0.871429 -0.857143 -0.842857 -0.828571 -0.814286 -0.8 -0.785714 -0.771429 -0.757143 -0.742857 -0.728571 -0.714286 -0.7 -0.685714 -0.671429 -0.657143 -0.642857 -0.628571 -0.614286 -0.6 -0.585714 -0.571429 -0.557143 -0.542857 -0.528571 -0.514286 -0.5 -0.485714 -0.471429 -0.457143 -0.442857 -0.428571 -0.414286 -0.4 -0.385714 -0.371429 -0.357143 -0.354152 -0.354152 -0.354152 -0.354152 -0.354152 -0.354152
  spline S23 degree 3 poles (-67.1352, -14.4636) (-67.1658, -14.4062) (-67.2073, -14.3552) (-67.3076, -14.2722) (-67.3654, -14.2409) (-67.4687, -14.2086) (-67.5113, -14.2012) (-67.5975, -14.1974) (-67.6406, -14.2011) (-67.6827, -14.2102) knots 0 0 0 0 0.019532 0.019532 0.039064 0.039064 0.051994 0.051994 0.064924 0.064924 0.064924 0.064924
  arc A12 (-67.1352, -14.4636) -> (-67.0952, -14.5383) centre (-40, 0) ccw
  spline S24 degree 3 poles (-67.1885, -15.1344) (-67.1416, -15.0892) (-67.1041, -15.0352) (-67.0518, -14.916) (-67.0375, -14.8518) (-67.0349, -14.7436) (-67.0394, -14.7006) (-67.0594, -14.6168) (-67.0748, -14.5763) (-67.0952, -14.5383) knots 0 0 0 0 0.019532 0.019532 0.039064 0.039064 0.051994 0.051994 0.064924 0.064924 0.064924 0.064924
  spline S25 degree 5 poles (-67.1885, -15.1344) (-67.1898, -15.1357) (-67.1973, -15.143) (-67.2111, -15.1563) (-67.2311, -15.1758) (-67.2573, -15.2016) (-67.2882, -15.2323) (-67.319, -15.2632) (-67.3496, -15.2943) (-67.3802, -15.3256) (-67.4106, -15.3571) (-67.4409, -15.3887) (-67.471, -15.4205) (-67.5011, -15.4525) (-67.531, -15.4846) (-67.5608, -15.517) (-67.5905, -15.5494) (-67.6201, -15.5821) (-67.6495, -15.6149) (-67.6789, -15.6478) (-67.7081, -15.681) (-67.7372, -15.7142) (-67.7662, -15.7477) (-67.7951, -15.7812) (-67.8239, -15.8149) (-67.8526, -15.8488) (-67.8811, -15.8828) (-67.9096, -15.917) (-67.9379, -15.9513) (-67.9661, -15.9857) (-67.9943, -16.0203) (-68.0223, -16.055) (-68.0502, -16.0899) (-68.078, -16.1249) (-68.1057, -16.16) (-68.1333, -16.1953) (-68.1608, -16.2307) (-68.1882, -16.2662) (-68.2155, -16.3019) (-68.2427, -16.3377) (-68.2697, -16.3736) (-68.2967, -16.4096) (-68.3236, -16.4458) (-68.3504, -16.4821) (-68.377, -16.5185) (-68.4036, -16.5551) (-68.4301, -16.5917) (-68.4512, -16.6212) (-68.4669, -16.6433) (-68.4774, -16.6581) (-68.4827, -16.6655) knots 0.354152 0.354152 0.354152 0.354152 0.354152 0.354152 0.357143 0.371429 0.385714 0.4 0.414286 0.428571 0.442857 0.457143 0.471429 0.485714 0.5 0.514286 0.528571 0.542857 0.557143 0.571429 0.585714 0.6 0.614286 0.628571 0.642857 0.657143 0.671429 0.685714 0.7 0.714286 0.728571 0.742857 0.757143 0.771429 0.785714 0.8 0.814286 0.828571 0.842857 0.857143 0.871429 0.885714 0.9 0.914286 0.928571 0.942857 0.957143 0.971429 0.985714 1 1 1 1 1 1
  arc A13 (-68.4827, -16.6655) -> (-68.1167, -17.2757) centre (-40, 0) ccw
  spline S26 degree 5 poles (-68.1167, -17.2757) (-68.1077, -17.2746) (-68.0897, -17.2723) (-68.0628, -17.2688) (-68.0269, -17.264) (-67.9821, -17.258) (-67.9373, -17.2517) (-67.8927, -17.2454) (-67.848, -17.2388) (-67.8035, -17.2322) (-67.759, -17.2253) (-67.7145, -17.2184) (-67.6701, -17.2113) (-67.6258, -17.204) (-67.5816, -17.1966) (-67.5374, -17.189) (-67.4933, -17.1812) (-67.4493, -17.1734) (-67.4053, -17.1653) (-67.3614, -17.1571) (-67.3176, -17.1487) (-67.2738, -17.1402) (-67.2301, -17.1315) (-67.1865, -17.1227) (-67.143, -17.1137) (-67.0995, -17.1045) (-67.0562, -17.0952) (-67.0129, -17.0857) (-66.9696, -17.076) (-66.9265, -17.0661) (-66.8834, -17.0561) (-66.8405, -17.0459) (-66.7976, -17.0356) (-66.7548, -17.025) (-66.712, -17.0143) (-66.6694, -17.0034) (-66.6268, -16.9924) (-66.5844, -16.9811) (-66.542, -16.9697) (-66.4998, -16.9581) (-66.4576, -16.9462) (-66.4155, -16.9342) (-66.3735, -16.922) (-66.3316, -16.9096) (-66.2899, -16.897) (-66.2482, -16.8842) (-66.2132, -16.8733) (-66.1866, -16.8648) (-66.1683, -16.859) (-66.1583, -16.8557) (-66.1565, -16.8552) knots -1 -1 -1 -1 -1 -1 -0.985714 -0.971429 -0.957143 -0.942857 -0.928571 -0.914286 -0.9 -0.885714 -0.871429 -0.857143 -0.842857 -0.828571 -0.814286 -0.8 -0.785714 -0.771429 -0.757143 -0.742857 -0.728571 -0.714286 -0.7 -0.685714 -0.671429 -0.657143 -0.642857 -0.628571 -0.614286 -0.6 -0.585714 -0.571429 -0.557143 -0.542857 -0.528571 -0.514286 -0.5 -0.485714 -0.471429 -0.457143 -0.442857 -0.428571 -0.414286 -0.4 -0.385714 -0.371429 -0.357143 -0.354152 -0.354152 -0.354152 -0.354152 -0.354152 -0.354152
  spline S27 degree 3 poles (-65.5868, -17.0537) (-65.6229, -16.9995) (-65.6693, -16.9529) (-65.7772, -16.8801) (-65.8378, -16.8546) (-65.9437, -16.8326) (-65.9869, -16.8294) (-66.073, -16.8341) (-66.1155, -16.8419) (-66.1565, -16.8552) knots 0 0 0 0 0.019532 0.019532 0.039064 0.039064 0.051994 0.051994 0.064924 0.064924 0.064924 0.064924
  arc A14 (-65.5868, -17.0537) -> (-65.5397, -17.1241) centre (-40, 0) ccw
  spline S28 degree 3 poles (-65.5741, -17.7265) (-65.5319, -17.6769) (-65.4998, -17.6195) (-65.4595, -17.4957) (-65.4516, -17.4304) (-65.4596, -17.3225) (-65.4683, -17.2801) (-65.4965, -17.1987) (-65.5157, -17.1599) (-65.5397, -17.1241) knots 0 0 0 0 0.019532 0.019532 0.039064 0.039064 0.051994 0.051994 0.064924 0.064924 0.064924 0.064924
  spline S29 degree 5 poles (-65.5741, -17.7265) (-65.5753, -17.7278) (-65.5821, -17.7359) (-65.5945, -17.7505) (-65.6125, -17.7719) (-65.636, -17.8) (-65.6638, -17.8337) (-65.6914, -17.8674) (-65.7188, -17.9014) (-65.7461, -17.9355) (-65.7733, -17.9698) (-65.8004, -18.0043) (-65.8273, -18.0389) (-65.854, -18.0737) (-65.8807, -18.1086) (-65.9072, -18.1437) (-65.9335, -18.1789) (-65.9598, -18.2143) (-65.9859, -18.2498) (-66.0118, -18.2855) (-66.0377, -18.3213) (-66.0634, -18.3573) (-66.089, -18.3934) (-66.1144, -18.4296) (-66.1398, -18.466) (-66.165, -18.5025) (-66.1901, -18.5392) (-66.215, -18.576) (-66.2399, -18.6129) (-66.2646, -18.6499) (-66.2892, -18.6871) (-66.3137, -18.7244) (-66.338, -18.7618) (-66.3623, -18.7994) (-66.3864, -18.837) (-66.4104, -18.8748) (-66.4343, -18.9128) (-66.4581, -18.9508) (-66.4817, -18.989) (-66.5053, -19.0273) (-66.5287, -19.0657) (-66.552, -19.1042) (-66.5752, -19.1428) (-66.5983, -19.1815) (-66.6213, -19.2204) (-66.6441, -19.2594) (-66.6669, -19.2985) (-66.685, -19.3298) (-66.6985, -19.3534) (-66.7075, -19.3691) (-66.712, -19.377) knots 0.354152 0.354152 0.354152 0.354152 0.354152 0.354152 0.357143 0.371429 0.385714 0.4 0.414286 0.428571 0.442857 0.457143 0.471429 0.485714 0.5 0.514286 0.528571 0.542857 0.557143 0.571429 0.585714 0.6 0.614286 0.628571 0.642857 0.657143 0.671429 0.685714 0.7 0.714286 0.728571 0.742857 0.757143 0.771429 0.785714 0.8 0.814286 0.828571 0.842857 0.857143 0.871429 0.885714 0.9 0.914286 0.928571 0.942857 0.957143 0.971429 0.985714 1 1 1 1 1 1
  arc A15 (-66.712, -19.377) -> (-66.288, -19.9484) centre (-40, 0) ccw
  spline S30 degree 5 poles (-66.288, -19.9484) (-66.2792, -19.9464) (-66.2615, -19.9424) (-66.235, -19.9363) (-66.1998, -19.928) (-66.1558, -19.9176) (-66.1118, -19.907) (-66.068, -19.8963) (-66.0242, -19.8854) (-65.9805, -19.8744) (-65.9369, -19.8633) (-65.8934, -19.852) (-65.8499, -19.8405) (-65.8065, -19.8289) (-65.7632, -19.8172) (-65.72, -19.8053) (-65.6769, -19.7933) (-65.6338, -19.7812) (-65.5908, -19.7688) (-65.548, -19.7564) (-65.5052, -19.7438) (-65.4625, -19.731) (-65.4198, -19.7181) (-65.3773, -19.705) (-65.3349, -19.6917) (-65.2925, -19.6784) (-65.2503, -19.6648) (-65.2081, -19.6511) (-65.166, -19.6372) (-65.1241, -19.6232) (-65.0822, -19.609) (-65.0404, -19.5947) (-64.9987, -19.5802) (-64.9572, -19.5655) (-64.9157, -19.5506) (-64.8743, -19.5356) (-64.8331, -19.5204) (-64.7919, -19.5051) (-64.7509, -19.4895) (-64.71, -19.4738) (-64.6692, -19.4579) (-64.6285, -19.4419) (-64.5879, -19.4256) (-64.5474, -19.4092) (-64.5071, -19.3925) (-64.4669, -19.3757) (-64.4331, -19.3614) (-64.4074, -19.3504) (-64.3898, -19.3427) (-64.3802, -19.3385) (-64.3785, -19.3378) knots -1 -1 -1 -1 -1 -1 -0.985714 -0.971429 -0.957143 -0.942857 -0.928571 -0.914286 -0.9 -0.885714 -0.871429 -0.857143 -0.842857 -0.828571 -0.814286 -0.8 -0.785714 -0.771429 -0.757143 -0.742857 -0.728571 -0.714286 -0.7 -0.685714 -0.671429 -0.657143 -0.642857 -0.628571 -0.614286 -0.6 -0.585714 -0.571429 -0.557143 -0.542857 -0.528571 -0.514286 -0.5 -0.485714 -0.471429 -0.457143 -0.442857 -0.428571 -0.414286 -0.4 -0.385714 -0.371429 -0.357143 -0.354152 -0.354152 -0.354152 -0.354152 -0.354152 -0.354152
  spline S31 degree 3 poles (-63.7921, -19.4795) (-63.8333, -19.4291) (-63.884, -19.3873) (-63.9986, -19.3254) (-64.0613, -19.3059) (-64.1689, -19.2945) (-64.2122, -19.2955) (-64.2974, -19.3086) (-64.339, -19.3206) (-64.3785, -19.3378) knots 0 0 0 0 0.019532 0.019532 0.039064 0.039064 0.051994 0.051994 0.064924 0.064924 0.064924 0.064924
  arc A16 (-63.7921, -19.4795) -> (-63.7383, -19.545) centre (-40, 0) ccw
  spline S32 degree 3 poles (-63.7135, -20.1478) (-63.6764, -20.0943) (-63.65, -20.0341) (-63.622, -19.9069) (-63.6205, -19.8412) (-63.6391, -19.7346) (-63.6519, -19.6933) (-63.6879, -19.6149) (-63.7109, -19.5783) (-63.7383, -19.545) knots 0 0 0 0 0.019532 0.019532 0.039064 0.039064 0.051994 0.051994 0.064924 0.064924 0.064924 0.064924
  spline S33 degree 5 poles (-63.7135, -20.1478) (-63.7145, -20.1493) (-63.7205, -20.1579) (-63.7314, -20.1737) (-63.7472, -20.1968) (-63.7678, -20.2271) (-63.7922, -20.2633) (-63.8163, -20.2996) (-63.8403, -20.3361) (-63.8642, -20.3727) (-63.8879, -20.4095) (-63.9114, -20.4465) (-63.9348, -20.4835) (-63.958, -20.5208) (-63.9811, -20.5581) (-64.004, -20.5957) (-64.0268, -20.6333) (-64.0494, -20.6711) (-64.0719, -20.709) (-64.0943, -20.7471) (-64.1165, -20.7852) (-64.1385, -20.8235) (-64.1605, -20.862) (-64.1823, -20.9005) (-64.2039, -20.9392) (-64.2254, -20.978) (-64.2468, -21.017) (-64.268, -21.056) (-64.2891, -21.0952) (-64.3101, -21.1345) (-64.331, -21.1739) (-64.3517, -21.2134) (-64.3722, -21.2531) (-64.3927, -21.2928) (-64.413, -21.3327) (-64.4332, -21.3726) (-64.4533, -21.4127) (-64.4732, -21.4529) (-64.493, -21.4932) (-64.5127, -21.5336) (-64.5322, -21.5741) (-64.5516, -21.6147) (-64.5709, -21.6555) (-64.5901, -21.6963) (-64.6092, -21.7372) (-64.6281, -21.7782) (-64.6469, -21.8193) (-64.6619, -21.8523) (-64.673, -21.8771) (-64.6804, -21.8936) (-64.6841, -21.9019) knots 0.354152 0.354152 0.354152 0.354152 0.354152 0.354152 0.357143 0.371429 0.385714 0.4 0.414286 0.428571 0.442857 0.457143 0.471429 0.485714 0.5 0.514286 0.528571 0.542857 0.557143 0.571429 0.585714 0.6 0.614286 0.628571 0.642857 0.657143 0.671429 0.685714 0.7 0.714286 0.728571 0.742857 0.757143 0.771429 0.785714 0.8 0.814286 0.828571 0.842857 0.857143 0.871429 0.885714 0.9 0.914286 0.928571 0.942857 0.957143 0.971429 0.985714 1 1 1 1 1 1
  arc A17 (-64.6841, -21.9019) -> (-64.2061, -22.4291) centre (-40, 0) ccw
  spline S34 degree 5 poles (-64.2061, -22.4291) (-64.1975, -22.4262) (-64.1804, -22.4204) (-64.1546, -22.4117) (-64.1203, -22.4001) (-64.0776, -22.3854) (-64.0349, -22.3705) (-63.9923, -22.3556) (-63.9498, -22.3405) (-63.9074, -22.3252) (-63.8651, -22.3099) (-63.8229, -22.2944) (-63.7807, -22.2787) (-63.7387, -22.2629) (-63.6967, -22.247) (-63.6549, -22.231) (-63.6131, -22.2148) (-63.5715, -22.1985) (-63.5299, -22.182) (-63.4885, -22.1654) (-63.4471, -22.1486) (-63.4059, -22.1317) (-63.3647, -22.1147) (-63.3237, -22.0975) (-63.2827, -22.0802) (-63.2419, -22.0627) (-63.2012, -22.0451) (-63.1606, -22.0273) (-63.1201, -22.0094) (-63.0797, -21.9913) (-63.0394, -21.9731) (-62.9992, -21.9547) (-62.9592, -21.9362) (-62.9192, -21.9175) (-62.8794, -21.8987) (-62.8397, -21.8797) (-62.8002, -21.8605) (-62.7607, -21.8412) (-62.7214, -21.8217) (-62.6822, -21.8021) (-62.6432, -21.7822) (-62.6042, -21.7623) (-62.5654, -21.7421) (-62.5268, -21.7218) (-62.4883, -21.7013) (-62.4499, -21.6806) (-62.4177, -21.663) (-62.3932, -21.6495) (-62.3764, -21.6402) (-62.3673, -21.6351) (-62.3657, -21.6342) knots -1 -1 -1 -1 -1 -1 -0.985714 -0.971429 -0.957143 -0.942857 -0.928571 -0.914286 -0.9 -0.885714 -0.871429 -0.857143 -0.842857 -0.828571 -0.814286 -0.8 -0.785714 -0.771429 -0.757143 -0.742857 -0.728571 -0.714286 -0.7 -0.685714 -0.671429 -0.657143 -0.642857 -0.628571 -0.614286 -0.6 -0.585714 -0.571429 -0.557143 -0.542857 -0.528571 -0.514286 -0.5 -0.485714 -0.471429 -0.457143 -0.442857 -0.428571 -0.414286 -0.4 -0.385714 -0.371429 -0.357143 -0.354152 -0.354152 -0.354152 -0.354152 -0.354152 -0.354152
  spline S35 degree 3 poles (-61.7682, -21.7177) (-61.8141, -21.6717) (-61.8687, -21.635) (-61.9888, -21.5846) (-62.0532, -21.5714) (-62.1614, -21.5706) (-62.2043, -21.5758) (-62.2878, -21.5972) (-62.328, -21.6132) (-62.3657, -21.6342) knots 0 0 0 0 0.019532 0.019532 0.039064 0.039064 0.051994 0.051994 0.064924 0.064924 0.064924 0.064924
  arc A18 (-61.7682, -21.7177) -> (-61.7082, -21.7776) centre (-40, 0) ccw
  spline S36 degree 3 poles (-61.6244, -22.3751) (-61.5928, -22.3182) (-61.5725, -22.2557) (-61.557, -22.1264) (-61.562, -22.0609) (-61.5909, -21.9566) (-61.6078, -21.9167) (-61.6513, -21.8423) (-61.6777, -21.8081) (-61.7082, -21.7776) knots 0 0 0 0 0.019532 0.019532 0.039064 0.039064 0.051994 0.051994 0.064924 0.064924 0.064924 0.064924